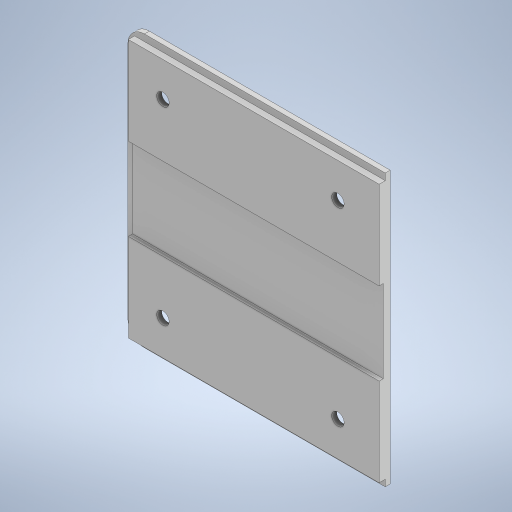
# Autodesk Inventor part: SlaveLåg
Saved by Autodesk Inventor 2023 (Build 270158000, 158)
## iProperties
Created: 2023-12-06
Part Number: SlaveLåg
Material: Generic
Document SubType Name: Modeling
Designer: Bruger
Density: 1 g/cm^3
Appearance: Default
Author: Bruger
Autodesk Inventor part; units mm, degrees
ref_plane "YZ Plane" through (0, 0, 0) normal (1, 0, 0) x (0, 1, 0)
ref_plane "XZ Plane" through (0, 0, 0) normal (0, 1, 0) x (-1, 0, 0)
ref_plane "XY Plane" through (0, 0, 0) normal (0, 0, 1) x (1, 0, 0)
sketch "Sketch1" plane through (0, 0, 0) normal (0, 0, 1) x (1, 0, 0)
  line L0 (0, 0) -> (62.5, 0)
  line L1 (62.5, 0) -> (62.5, 66)
  line L2 (62.5, 66) -> (0, 66)
  line L3 (0, 66) -> (0, 0)
  dimension "d0" = 62.5
  dimension "d1" = 66
  constraints: 8 end point, 2 parallel, 1 horizontal, 1 perpendicular
  measures "d0" distance of L2.end L1.end
  measures "d1" distance of L1.end L0.end
extrude "Extrusion1" add sketch "Sketch1" along normal blind 1.2
sketch "Sketch2" plane through (0, 0, 1.2) normal (0, 0, 1) x (1, 0, 0)
  line L0 (62.5, 66) -> (0, 66) projected
  line L1 (0, 66) -> (0, 0) projected
  line L2 (62.5, 66) -> (0, 66)
  line L3 (0, 66) -> (0, 64.4)
  line L4 (0, 64.4) -> (62.5, 64.4)
  line L5 (62.5, 64.4) -> (62.5, 66)
  line L6 (62.5, 0) -> (62.5, 66) projected
  line L7 (62.5, 0) -> (0, 0)
  line L8 (0, 0) -> (0, 1.6)
  line L9 (0, 1.6) -> (62.5, 1.6)
  line L10 (62.5, 1.6) -> (62.5, 0)
  line L11 (0, 0) -> (62.5, 0) projected
  line L12 (0, 66) -> (1.6, 66)
  line L13 (1.6, 66) -> (1.6, 0)
  line L14 (1.6, 0) -> (0, 0)
  line L15 (0, 0) -> (0, 66)
  line L16 (62.5, 64.4) -> (1.6, 64.4)
  line L17 (1.6, 64.4) -> (1.6, 1.6)
  line L18 (1.6, 1.6) -> (62.5, 1.6)
  line L19 (62.5, 1.6) -> (62.5, 64.4)
  dimension "d4" = 1.6
  dimension "d5" = 1.6
  dimension "d6" = 1.6
  constraints: 32 end point, 8 parallel, 5 point on line, 4 horizontal, 4 perpendicular
  measures "d4" distance of L3.end L2.end
  measures "d5" distance of L7.end L8.end
  measures "d6" distance of L13.end L14.end
extrude "Extrusion2" add sketch "Sketch2" along normal blind 1.5 contours L6 L9 L13 L4
sketch "Sketch3" plane through (0, 0, 2.7) normal (0, 0, 1) x (1, 0, 0)
  line L0 (1.6, 1.6) -> (1.6, 64.4) projected
  line L1 (1.6, 1.6) -> (1.6, 64.4)
  line L2 (1.6, 33) -> (1.6, 43)
  line L3 (1.6, 43) -> (64.8797, 43)
  line L4 (64.8797, 43) -> (64.8797, 23)
  line L5 (64.8797, 23) -> (1.6, 23)
  line L6 (1.6, 23) -> (1.6, 43)
  point P0 (0, 0)
  point P1 (1.6, 23)
  dimension "d9" = 10
  dimension "d10" = 20
  constraints: 12 end point, 3 equal length, 1 horizontal, 1 midpoint, 1 perpendicular, 1 point on line
  measures "d9" distance of L2.start L2.end
  measures "d10" distance of L3.end L4.end
extrude "Extrusion3" cut sketch "Sketch3" against normal blind 1
sketch "Sketch4" plane through (0, 0, 2.7) normal (0, 0, 1) x (1, 0, 0)
  line L0 (62.5, 64.4) -> (1.6, 64.4) projected
  line L1 (62.5, 1.6) -> (1.6, 1.6) projected
  line L2 (1.6, 64.4) -> (60.9, 64.4)
  line L3 (60.9, 64.4) -> (60.9, 1.6)
  line L4 (60.9, 1.6) -> (1.6, 1.6)
  line L5 (1.6, 1.6) -> (1.6, 64.4)
  line L6 (0, 66) -> (0, 0) projected
  circle A0 centre (10, 56) radius 1.5
  line L7 (62.5, 0) -> (62.5, 66) projected
  circle A1 centre (52.5, 56) radius 1.5
  circle A2 centre (10, 10) radius 1.5
  circle A3 centre (52.5, 10) radius 1.5
  dimension "d13" = 59.3
  constraints: 8 end point, 4 centre point, 2 parallel, 1 horizontal, 1 perpendicular, 1 point on line
  measures "d13" distance of L3.end L4.end
extrude "Extrusion4" cut sketch "Sketch4" against normal through all contours A0 | A1 | A2 | A3
sketch "Sketch5" plane through (0, 0, 0) normal (0, 0, -1) x (-1, 0, 0)
  circle A0 centre (-52.5, 56) radius 1.5 projected
  circle A1 centre (-52.5, 56) radius 6
  circle A2 centre (-10, 56) radius 1.5 projected
  circle A3 centre (-10, 56) radius 6
  circle A4 centre (-52.5, 10) radius 1.5 projected
  circle A5 centre (-52.5, 10) radius 6
  circle A6 centre (-10, 10) radius 1.5 projected
  circle A7 centre (-10, 10) radius 6.5
  point P0 (0, 0)
  dimension "d22" = 12
  dimension "d23" = 12
  dimension "d24" = 12
  dimension "d25" = 13
  constraints: 4 centre point, 4 coincident
  measures "d22" diameter of A1
  measures "d23" diameter of A3
  measures "d24" diameter of A5
  measures "d25" diameter of A7
extrude "Extrusion5" cut sketch "Sketch5" against normal blind 1.5 contours A0 | A1 | A3 | A4 | A5 | A7
fillet "Fillet1" radius 4 2 edges at (0, 66, 0.6) (0, 0, 0.6)
body "Solid1"
